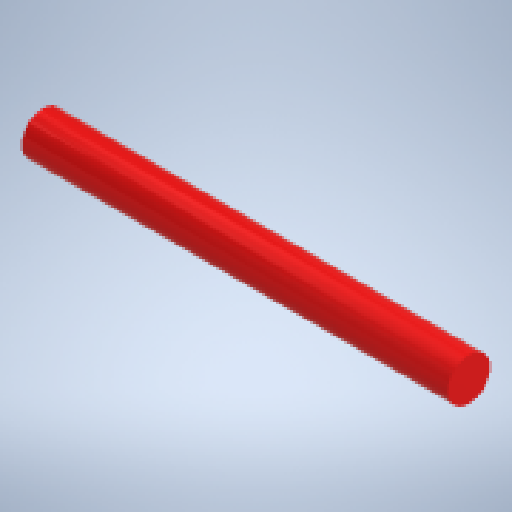
# Autodesk Inventor part: Thermistor
Saved by Autodesk Inventor 2025.3 (Build 293356000, 356)
## iProperties
Created: 2025-05-19
Part Number: Thermistor
Material: Genérico
Document SubType Name: Modeling
Designer: dell 5810
Density: 1 g/cm^3
Appearance: Suave - Rojo
Author: dell 5810
Autodesk Inventor part; units mm, degrees
ref_plane "YZ Plane" through (0, 0, 0) normal (1, 0, 0) x (0, 1, 0)
ref_plane "XZ Plane" through (0, 0, 0) normal (0, 1, 0) x (-1, 0, 0)
ref_plane "XY Plane" through (0, 0, 0) normal (0, 0, 1) x (1, 0, 0)
sketch "Boceto1" plane through (0, 0, 0) normal (1, 0, 0) x (0, 1, 0)
  circle A0 centre (0, 0) radius 0.5
  dimension "d0" = 1
  constraints: 1 centre point, 1 coincident
  measures "d0" diameter of A0
extrude "Extrusión1" add sketch "Boceto1" along normal blind 10
sketch "Boceto2" plane through (10, 0, 0) normal (1, 0, 0) x (0, 0, -1)
  circle A0 centre (0, 0) radius 0.5 projected
sketch "Sketch3" plane through (0, 0, 0) normal (-1, 0, 0) x (0, 0, 1)
  circle A0 centre (0, 0) radius 0.5 projected
sketch "Sketch4" plane through (10, 0, 0) normal (1, 0, 0) x (0, 0, -1)
  circle A0 centre (0, 0) radius 0.5 projected
